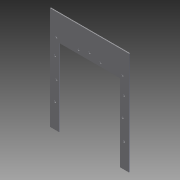
# Autodesk Inventor part: top mid-pivot plate
Saved by Autodesk Inventor 2011 SP1 (Build 150282100, 282)
## iProperties
Created: 2012-01-20
Part Number: top mid-pivot plate
Document SubType Name: Modeling
Designer: Christopher
Density: 1 g/cm^3
Author: Christopher
Autodesk Inventor part; units mm, degrees
ref_plane "YZ Plane" through (0, 0, 0) normal (1, 0, 0) x (0, 1, 0)
ref_plane "XZ Plane" through (0, 0, 0) normal (0, 1, 0) x (-1, 0, 0)
ref_plane "XY Plane" through (0, 0, 0) normal (0, 0, 1) x (1, 0, 0)
sketch "Sketch1" plane through (0, 0, 0) normal (0, 0, 1) x (1, 0, 0)
  line L0 (333.7348, 152.4) -> (333.7348, 508)
  line L1 (92.4348, 152.4) -> (92.4348, 419.1)
  line L2 (92.4348, 419.1) -> (301.9848, 419.1)
  line L3 (301.9848, 419.1) -> (301.9848, 152.4)
  line L4 (301.9848, 152.4) -> (333.7348, 152.4)
  line L5 (92.4348, 152.4) -> (60.6848, 152.4)
  line L6 (60.6848, 152.4) -> (60.6848, 508)
  line L7 (333.7348, 508) -> (60.6848, 508)
  point P0 (0, 0)
  point P1 (197.2098, 304.8)
  point P2 (197.2098, 442.341)
  point P3 (78.0958, 373.5705)
  point P4 (78.0958, 236.0295)
  point P5 (197.2098, 167.259)
  point P6 (316.3238, 236.0295)
  point P7 (316.3238, 373.5705)
  point P8 (311.5098, 304.8)
  point P9 (311.5098, 431.8)
  point P10 (82.9098, 431.8)
  point P11 (82.9098, 304.8)
  point P12 (235.3098, 431.8)
  point P13 (159.1098, 431.8)
  dimension "d1" = 355.6
  dimension "d4" = 137.541
  dimension "d7" = 360
  dimension "d9" = 31.75
  dimension "d21" = 31.75
  dimension "d23" = 114.3
  dimension "d39" = 127
  dimension "d40" = 127
  dimension "d48" = 22.225
  dimension "d49" = 22.225
  dimension "d54" = 209.55
  dimension "d55" = 266.7
  dimension "d56" = 104.775
  dimension "d57" = 152.4
  dimension "d58" = 152.4
  constraints: 16 end point, 4 perpendicular, 3 horizontal alignment, 2 vertical alignment, 1 collinear, 7 other
  measures "d1" distance of L0.end L0.start
  measures "d4" distance of point (197.21, 442.341) point (197.21, 304.8)
  measures "d9" distance between parallel lines of L0 L3
  measures "d21" distance of L1.start L5.end
  measures "d23" distance from line of point (197.21, 304.8) L2
  measures "d39" distance of point (311.51, 304.8) point (311.51, 431.8)
  measures "d40" distance of point (82.91, 431.8) point (82.91, 304.8)
  measures "d48" distance from line of L6 point (82.91, 431.8)
  measures "d49" distance from line of L0 point (311.51, 431.8)
  measures "d54" distance of L1.end L2.end
  measures "d55" distance of L2.end L3.end
  measures "d56" distance from line of L1 point (197.21, 304.8)
  measures "d57" distance from line of L4 point (311.51, 304.8)
  measures "d58" distance from line of L5 point (82.91, 304.8)
extrude "Extrusion1" add sketch "Sketch1" against normal blind 3.175
hole "Hole1" at (197.2098, 304.8, 0) at (197.2098, 442.341, 0) at (78.0958, 373.5705, 0) at (78.0958, 236.0295, 0) at (197.2098, 167.259, 0) at (316.3238, 236.0295, 0) at (316.3238, 373.5705, 0) direction (0, 0, -1) diameter 6.35 depth 25.4 tip angle 118
hole "Hole3" at (311.5098, 304.8, 0) at (311.5098, 431.8, 0) at (82.9098, 431.8, 0) at (82.9098, 304.8, 0) at (159.1098, 431.8, 0) at (235.3098, 431.8, 0) direction (0, 0, -1) diameter 6.35 depth 25.4 tip angle 118
body "Solid1"
